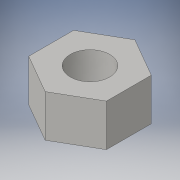
# Autodesk Inventor part: 10-32 nut
Saved by Autodesk Inventor 2016 (Build 200138000, 138)
## iProperties
Created: 2016-01-17
Part Number: 10-32 nut
Material: Generic
Document SubType Name: Modeling
Designer: gus
Density: 1 g/cm^3
Appearance: Default
Author: gus
Autodesk Inventor part; units mm, degrees
ref_plane "YZ Plane" through (0, 0, 0) normal (1, 0, 0) x (0, 1, 0)
ref_plane "XZ Plane" through (0, 0, 0) normal (0, 1, 0) x (-1, 0, 0)
ref_plane "XY Plane" through (0, 0, 0) normal (0, 0, 1) x (1, 0, 0)
sketch "Sketch1" plane through (0, 0, 0) normal (0, 1, 0) x (-1, 0, 0)
  circle A0 centre (0, 0) radius 2.413
  line L0 (4.7625, -2.7496) -> (0, -5.4993)
  line L1 (0, -5.4993) -> (-4.7625, -2.7496)
  line L2 (-4.7625, -2.7496) -> (-4.7625, 2.7496)
  line L3 (-4.7625, 2.7496) -> (0, 5.4993)
  line L4 (0, 5.4993) -> (4.7625, 2.7496)
  line L5 (4.7625, 2.7496) -> (4.7625, -2.7496)
  dimension "d0" = 4.826
  dimension "d1" = 9.525
  constraints: 12 end point, 2 coincident, 1 centre point, 1 vertical, 13 other
  measures "d0" diameter of A0
  measures "d1" distance between parallel lines of L5 L2
extrude "Extrusion1" add sketch "Sketch1" along normal blind 5.1562
body "Solid1"
